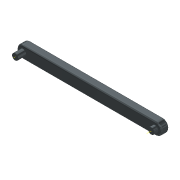
# Autodesk Inventor part: Acoplador
Saved by Autodesk Inventor 2021 (Build 250183000, 183)
## iProperties
Created: 2021-07-04
Part Number: Acoplador
Material: Iron, Ductile
Document SubType Name: Modeling
Designer: Santiago
Density: 7.15 g/cm^3
Appearance: Iron Gray
Mass: 209.491 g
Surface Area: 94.482 cm^2
Volume: 29.2994 cm^3
Author: Santiago
Autodesk Inventor part; units mm, degrees
ref_plane "XZ Plane" through (0, 0, 0) normal (0, 1, 0) x (-1, 0, 0)
ref_plane "XY Plane" through (0, 0, 0) normal (0, 0, 1) x (1, 0, 0)
sketch "Sketch1" plane through (0, 0, 0) normal (0, 0, 1) x (1, 0, 0)
  circle A0 centre (0, 0) radius 8
  dimension "d0" = 16
  constraints: 1 centre point, 1 coincident
  measures "d0" diameter of A0
extrude "Extrusion1" add sketch "Sketch1" along normal blind 10
ref_plane "Work Plane1" through (8, 0, 0) normal (1, 0, 0) x (0, 1, 0)
sketch "Sketch2" plane through (8, 0, 0) normal (1, 0, 0) x (0, 1, 0)
  line L0 (-8, 0) -> (-8, 10) projected
  line L1 (8, 10) -> (-8, 10)
  line L2 (-8, 10) -> (-8, 0)
  line L3 (-8, 0) -> (8, 0)
  line L4 (8, 0) -> (8, 10)
  line L5 (8, 10) -> (-8, 0) construction
  line L6 (-8, 10) -> (8, 0) construction
  point P0 (0, 0)
  point P1 (0, 5)
  constraints: 12 end point, 2 midpoint, 2 parallel, 1 horizontal, 1 perpendicular, 1 point on line
extrude "Extrusion2" add sketch "Sketch2" along normal blind 162 and the other way blind 8
sketch "Sketch3" plane through (0, 0, 10) normal (0, 0, 1) x (1, 0, 0)
  arc A0 (0, 8) -> (0, -8) centre (0, 0) ccw projected
  line L0 (0, 0) -> (170, 0)
  line L1 (170, -8) -> (0, -8) projected
  line L2 (0, 0) -> (170, 0) construction
  line L3 (170, 8) -> (170, -8) projected
  circle A1 centre (170, 0) radius 8
  dimension "d8" = 170
  dimension "d9" = 0
  constraints: 4 end point, 1 coincident, 1 collinear, 1 horizontal, 1 parallel, 1 vertical alignment, 2 other
  measures "d8" distance of L0.start L0.end
  measures "d9" distance between parallel lines of L0 L2
extrude "Extrusion3" add sketch "Sketch3" against normal blind 10
ref_plane "Work Plane2" through (-8, 0, 0) normal (1, 0, 0) x (0, 1, 0)
sketch "Sketch4" plane through (-8, 0, 0) normal (1, 0, 0) x (0, 1, 0)
  line L0 (-8, 0) -> (-8, 10) projected
  line L1 (8, 7.5) -> (-8, 7.5)
  line L2 (-8, 7.5) -> (-8, 2.5)
  line L3 (-8, 2.5) -> (8, 2.5)
  line L4 (8, 2.5) -> (8, 7.5)
  line L5 (8, 7.5) -> (-8, 2.5) construction
  line L6 (-8, 7.5) -> (8, 2.5) construction
  line L7 (8, 10) -> (-8, 10) projected
  line L8 (8, 0) -> (8, 10) projected
  line L9 (-8, 10) -> (-8, 0) projected
  line L10 (-8, 0) -> (8, 0) projected
  point P0 (0, 0)
  point P1 (0, 5)
  dimension "d13" = 5
  constraints: 12 end point, 2 midpoint, 2 parallel, 1 horizontal, 1 perpendicular, 1 point on line
  measures "d13" distance of L2.end L1.end
extrude "Extrusion4" [suppressed]
sketch "Sketch5" plane through (0, -8, 7.5) normal (0, 0, 1) x (1, 0, 0)
  circle A0 centre (0, 8) radius 4
  dimension "d16" = 8
  constraints: 1 centre point, 1 coincident
  measures "d16" diameter of A0
extrude "Extrusion5" [suppressed]
sketch "Sketch6" plane through (0, 0, 10) normal (0, 0, 1) x (1, 0, 0)
  arc A0 (170, -8) -> (170, 8) centre (170, 0) ccw projected
  circle A1 centre (170, 0) radius 4
  point P0 (0, 0)
  dimension "d21" = 8
  constraints: 1 centre point, 1 coincident
  measures "d21" diameter of A1
extrude "Extrusion6" add sketch "Sketch6" along normal blind 5
sketch "Sketch7" plane through (0, 0, 10) normal (0, 0, 1) x (1, 0, 0)
  circle A0 centre (0, 0) radius 4
  dimension "d24" = 8
  constraints: 1 centre point, 1 coincident
  measures "d24" diameter of A0
extrude "Extrusion7" add sketch "Sketch7" along normal blind 10
fillet "Fillet1" radius 2 8 edges at (178, 0, 0) (85, -8, 0) (-8, 0, 0) (85, 8, 0) (178, 0, 10) (85, -8, 10) (-8, 0, 10) (85, 8, 10)
body "Solid1"
